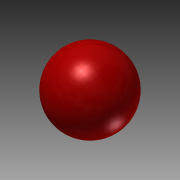
# Autodesk Inventor part: Ball
Saved by Autodesk Inventor 2014 (Build 180170000, 170)
## iProperties
Created: 2014-01-06
Part Number: Ball
Material: Generic
Document SubType Name: Modeling
Designer: Andrew Toennies
Density: 0.370967 g/cm^3
Appearance: Default
Mass: 1360.78 g
Surface Area: 23107.1 cm^2
Volume: 3668.19 cm^3
Author: Andrew Toennies
Autodesk Inventor part; units mm, degrees
ref_plane "YZ Plane" through (0, 0, 0) normal (1, 0, 0) x (0, 1, 0)
ref_plane "XZ Plane" through (0, 0, 0) normal (0, 1, 0) x (-1, 0, 0)
ref_plane "XY Plane" through (0, 0, 0) normal (0, 0, 1) x (1, 0, 0)
sketch "Sketch1" plane through (0, 0, 0) normal (0, 0, 1) x (1, 0, 0)
  arc A0 (0, -317.5) -> (0, 317.5) centre (0, 0) ccw
  arc A1 (0, -314.325) -> (0, 314.325) centre (0, 0) ccw
  line L0 (0, 421.0105) -> (0, -428.3933)
  dimension "d0" = 635
  dimension "d1" = 3.175
  constraints: 5 point on line, 4 point on circle, 2 centre point, 2 end point, 1 coincident, 1 vertical
  measures "d0" diameter of A0
  measures "d1" radial gap between concentric circles of A0 A1
revolve "Revolution1" add sketch "Sketch1" angle 360 about axis through (0, 421.0105, 0) along (0, -1, 0) contours L0 A1 A0
body "Solid1"
